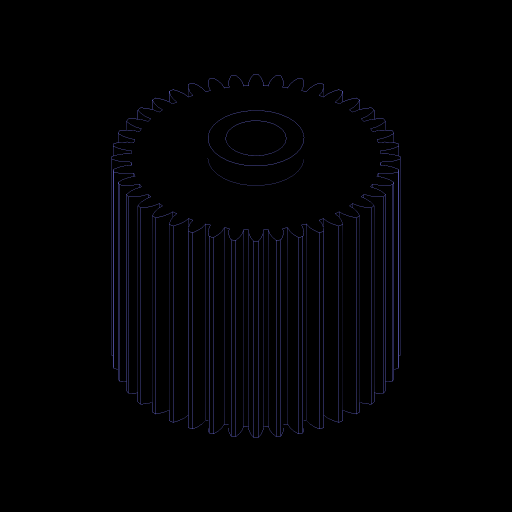
# Autodesk Inventor part: 피니언기어
Saved by Autodesk Inventor 2023 (Build 270158000, 158)
## iProperties
Created: 2024-07-04
Part Number: 피니언기어
Material: 일반
Document SubType Name: Modeling
Designer: OMS55
Density: 1 g/cm^3
Appearance: 기본값
Mass: 14.1026 g
Surface Area: 70.7702 cm^2
Volume: 14.1026 cm^3
Author: OMS55
Autodesk Inventor part; units mm, degrees
ref_plane "YZ Plane" through (0, 0, 0) normal (1, 0, 0) x (0, 1, 0)
ref_plane "XZ Plane" through (0, 0, 0) normal (0, 1, 0) x (-1, 0, 0)
ref_plane "XY Plane" through (0, 0, 0) normal (0, 0, 1) x (1, 0, 0)
sketch "스케치1" plane through (0, 0, 0) normal (0, 1, 0) x (-1, 0, 0)
  circle A0 centre (0, 0) radius 15
  arc A1 (12.978, 0.7559) -> (12.978, -0.7559) centre (0, 0) ccw
  line L0 (15, 0) -> (-15, 0) construction
  line L1 (14.9746, 0.8722) -> (-14.9746, -0.8722) construction
  line L2 (14.8986, 1.7414) -> (-14.8986, -1.7414) construction
  line L3 (14.7721, 2.6047) -> (-14.7721, -2.6047) construction
  line L4 (14.5957, 3.4592) -> (-14.5957, -3.4592) construction
  line L5 (14.3698, 4.302) -> (-14.3698, -4.302) construction
  line L6 (14.0954, 5.1303) -> (-14.0954, -5.1303) construction
  line L7 (13.7732, 5.9412) -> (-13.7732, -5.9412) construction
  line L8 (13.4045, 6.732) -> (-13.4045, -6.732) construction
  line L9 (12.9904, 7.5) -> (-12.9904, -7.5) construction
  line L10 (12.5323, 8.2426) -> (-12.5323, -8.2426) construction
  line L11 (12.0318, 8.9574) -> (-12.0318, -8.9574) construction
  line L12 (11.4907, 9.6418) -> (-11.4907, -9.6418) construction
  line L13 (10.9106, 10.2936) -> (-10.9106, -10.2936) construction
  line L14 (10.2936, 10.9106) -> (-10.2936, -10.9106) construction
  line L15 (9.6418, 11.4907) -> (-9.6418, -11.4907) construction
  line L16 (8.9574, 12.0318) -> (-8.9574, -12.0318) construction
  line L17 (8.2426, 12.5323) -> (-8.2426, -12.5323) construction
  line L18 (7.5, 12.9904) -> (-7.5, -12.9904) construction
  line L19 (6.732, 13.4045) -> (-6.732, -13.4045) construction
  line L20 (5.9412, 13.7732) -> (-5.9412, -13.7732) construction
  line L21 (5.1303, 14.0954) -> (-5.1303, -14.0954) construction
  line L22 (4.302, 14.3698) -> (-4.302, -14.3698) construction
  line L23 (3.4592, 14.5957) -> (-3.4592, -14.5957) construction
  line L24 (2.6047, 14.7721) -> (-2.6047, -14.7721) construction
  line L25 (1.7414, 14.8986) -> (-1.7414, -14.8986) construction
  line L26 (0.8722, 14.9746) -> (-0.8722, -14.9746) construction
  line L27 (0, 15) -> (0, -15) construction
  line L28 (-0.8722, 14.9746) -> (0.8722, -14.9746) construction
  line L29 (-1.7414, 14.8986) -> (1.7414, -14.8986) construction
  line L30 (-2.6047, 14.7721) -> (2.6047, -14.7721) construction
  line L31 (-3.4592, 14.5957) -> (3.4592, -14.5957) construction
  line L32 (-4.302, 14.3698) -> (4.302, -14.3698) construction
  line L33 (-5.1303, 14.0954) -> (5.1303, -14.0954) construction
  line L34 (-5.9412, 13.7732) -> (5.9412, -13.7732) construction
  line L35 (-6.732, 13.4045) -> (6.732, -13.4045) construction
  line L36 (-7.5, 12.9904) -> (7.5, -12.9904) construction
  line L37 (-8.2426, 12.5323) -> (8.2426, -12.5323) construction
  line L38 (-8.9574, 12.0318) -> (8.9574, -12.0318) construction
  line L39 (-9.6418, 11.4907) -> (9.6418, -11.4907) construction
  line L40 (-10.2936, 10.9106) -> (10.2936, -10.9106) construction
  line L41 (-10.9106, 10.2936) -> (10.9106, -10.2936) construction
  line L42 (-11.4907, 9.6418) -> (11.4907, -9.6418) construction
  line L43 (-12.0318, 8.9574) -> (12.0318, -8.9574) construction
  line L44 (-12.5323, 8.2426) -> (12.5323, -8.2426) construction
  line L45 (-12.9904, 7.5) -> (12.9904, -7.5) construction
  line L46 (-13.4045, 6.732) -> (13.4045, -6.732) construction
  line L47 (-13.7732, 5.9412) -> (13.7732, -5.9412) construction
  line L48 (-14.0954, 5.1303) -> (14.0954, -5.1303) construction
  line L49 (-14.3698, 4.302) -> (14.3698, -4.302) construction
  line L50 (-14.5957, 3.4592) -> (14.5957, -3.4592) construction
  line L51 (-14.7721, 2.6047) -> (14.7721, -2.6047) construction
  line L52 (-14.8986, 1.7414) -> (14.8986, -1.7414) construction
  line L53 (-14.9746, 0.8722) -> (14.9746, -0.8722) construction
  line L54 (-15, 0) -> (15, 0) construction
  line L55 (-14.9746, -0.8722) -> (14.9746, 0.8722) construction
  line L56 (-14.8986, -1.7414) -> (14.8986, 1.7414) construction
  line L57 (-14.7721, -2.6047) -> (14.7721, 2.6047) construction
  line L58 (-14.5957, -3.4592) -> (14.5957, 3.4592) construction
  line L59 (-14.3698, -4.302) -> (14.3698, 4.302) construction
  line L60 (-14.0954, -5.1303) -> (14.0954, 5.1303) construction
  line L61 (-13.7732, -5.9412) -> (13.7732, 5.9412) construction
  line L62 (-13.4045, -6.732) -> (13.4045, 6.732) construction
  line L63 (-12.9904, -7.5) -> (12.9904, 7.5) construction
  line L64 (-12.5323, -8.2426) -> (12.5323, 8.2426) construction
  line L65 (-12.0318, -8.9574) -> (12.0318, 8.9574) construction
  line L66 (-11.4907, -9.6418) -> (11.4907, 9.6418) construction
  line L67 (-10.9106, -10.2936) -> (10.9106, 10.2936) construction
  line L68 (-10.2936, -10.9106) -> (10.2936, 10.9106) construction
  line L69 (-9.6418, -11.4907) -> (9.6418, 11.4907) construction
  line L70 (-8.9574, -12.0318) -> (8.9574, 12.0318) construction
  line L71 (-8.2426, -12.5323) -> (8.2426, 12.5323) construction
  line L72 (-7.5, -12.9904) -> (7.5, 12.9904) construction
  line L73 (-6.732, -13.4045) -> (6.732, 13.4045) construction
  line L74 (-5.9412, -13.7732) -> (5.9412, 13.7732) construction
  line L75 (-5.1303, -14.0954) -> (5.1303, 14.0954) construction
  line L76 (-4.302, -14.3698) -> (4.302, 14.3698) construction
  line L77 (-3.4592, -14.5957) -> (3.4592, 14.5957) construction
  line L78 (-2.6047, -14.7721) -> (2.6047, 14.7721) construction
  line L79 (-1.7414, -14.8986) -> (1.7414, 14.8986) construction
  line L80 (-0.8722, -14.9746) -> (0.8722, 14.9746) construction
  line L81 (0, -15) -> (0, 15) construction
  line L82 (0.8722, -14.9746) -> (-0.8722, 14.9746) construction
  line L83 (1.7414, -14.8986) -> (-1.7414, 14.8986) construction
  line L84 (2.6047, -14.7721) -> (-2.6047, 14.7721) construction
  line L85 (3.4592, -14.5957) -> (-3.4592, 14.5957) construction
  line L86 (4.302, -14.3698) -> (-4.302, 14.3698) construction
  line L87 (5.1303, -14.0954) -> (-5.1303, 14.0954) construction
  line L88 (5.9412, -13.7732) -> (-5.9412, 13.7732) construction
  line L89 (6.732, -13.4045) -> (-6.732, 13.4045) construction
  line L90 (7.5, -12.9904) -> (-7.5, 12.9904) construction
  line L91 (8.2426, -12.5323) -> (-8.2426, 12.5323) construction
  line L92 (8.9574, -12.0318) -> (-8.9574, 12.0318) construction
  line L93 (9.6418, -11.4907) -> (-9.6418, 11.4907) construction
  line L94 (10.2936, -10.9106) -> (-10.2936, 10.9106) construction
  line L95 (10.9106, -10.2936) -> (-10.9106, 10.2936) construction
  line L96 (11.4907, -9.6418) -> (-11.4907, 9.6418) construction
  line L97 (12.0318, -8.9574) -> (-12.0318, 8.9574) construction
  line L98 (12.5323, -8.2426) -> (-12.5323, 8.2426) construction
  line L99 (12.9904, -7.5) -> (-12.9904, 7.5) construction
  line L100 (13.4045, -6.732) -> (-13.4045, 6.732) construction
  line L101 (13.7732, -5.9412) -> (-13.7732, 5.9412) construction
  line L102 (14.0954, -5.1303) -> (-14.0954, 5.1303) construction
  line L103 (14.3698, -4.302) -> (-14.3698, 4.302) construction
  line L104 (14.5957, -3.4592) -> (-14.5957, 3.4592) construction
  line L105 (14.7721, -2.6047) -> (-14.7721, 2.6047) construction
  line L106 (14.8986, -1.7414) -> (-14.8986, 1.7414) construction
  line L107 (14.9746, -0.8722) -> (-14.9746, 0.8722) construction
  arc A2 (14.9979, 0.25) -> (12.978, 0.7559) centre (13.1805, -2.7211) ccw
  arc A3 (12.978, -0.7559) -> (14.9979, -0.25) centre (13.1805, 2.7211) ccw
  dimension "d0" = 30
  dimension "d3" = 26
  dimension "d6" = 360
  dimension "d8" = 0.5
  dimension "d9" = 0.25
  constraints: 216 end point, 10 point on circle, 4 centre point, 3 point on line, 2 coincident, 2 tangent, 1 horizontal, 1 vertical alignment, 325 other
  measures "d0" diameter of A0
  measures "d3" diameter of A1
  measures "d8" distance of A3.end A2.start
  measures "d9" distance of A2.start L0.start
extrude "돌출1" add sketch "스케치1" along normal blind 25 contours A0 A3 A1 A2 picked at (-3.702, 3.2737)
pattern_circular "원형 패턴1" count 40 over 360 about axis through (0, 0, 0) along (0, 1, 0) of "돌출1"
sketch "스케치2" plane through (0, 25, 0) normal (0, 1, 0) x (1, 0, 0)
  circle A0 centre (0, 0) radius 3.15
  dimension "d15" = 6.3
  constraints: 1 centre point, 1 coincident
  measures "d15" diameter of A0
extrude "돌출2" cut sketch "스케치2" against normal blind 100
sketch "스케치3" plane through (0, 25, 0) normal (0, 1, 0) x (1, 0, 0)
  circle A0 centre (0, 0) radius 5
  circle A1 centre (0, 0) radius 3.15
  dimension "d18" = 10
  dimension "d19" = 6.3
  constraints: 2 centre point, 2 coincident
  measures "d18" diameter of A0
  measures "d19" diameter of A1
extrude "돌출3" add sketch "스케치3" along normal blind 2.5 and the other way blind 27.5
